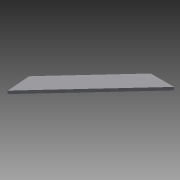
# Autodesk Inventor part: Ramp - End - Trapezoid Plywood 375
Saved by Autodesk Inventor 2015 (Build 190159000, 159)
## iProperties
Created: 2015-01-21
Part Number: Ramp - End - Trapezoid Plywood 375
Material: Generic
Document SubType Name: Modeling
Designer: peters
Density: 1 g/cm^3
Appearance: Default
Author: peters
Autodesk Inventor part; units mm, degrees
ref_plane "YZ Plane" through (0, 0, 0) normal (1, 0, 0) x (0, 1, 0)
ref_plane "XZ Plane" through (0, 0, 0) normal (0, 1, 0) x (-1, 0, 0)
ref_plane "XY Plane" through (0, 0, 0) normal (0, 0, 1) x (1, 0, 0)
sketch "Sketch1" plane through (0, 0, 0) normal (0, 1, 0) x (-1, 0, 0)
  line L0 (107.9233, 0) -> (299.9159, 207.4252)
  line L1 (299.9159, 207.4252) -> (291.5885, 315.0268)
  line L2 (291.5885, 315.0268) -> (0, 0)
  line L3 (0, 0) -> (107.9233, 0)
  line L4 (281.1686, 285.0731) -> (286.8255, 211.9789)
  line L5 (286.8255, 211.9789) -> (102.3731, 12.7)
  line L6 (102.3731, 12.7) -> (29.0604, 12.7)
  line L7 (29.0604, 12.7) -> (281.1686, 285.0731)
  point P0 (0, 0)
  dimension "d0" = 12.7
  constraints: 16 end point, 2 parallel, 1 horizontal, 3 other
  measures "d0" distance between parallel lines of L1 L4
extrude "Extrusion1" add sketch "Sketch1" along normal blind 9.525 contours L4 L5 L6 L7
body "Solid1"
